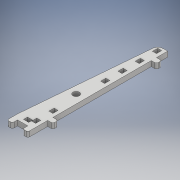
# Autodesk Inventor part: turtlebot_installation_fin_bottom
Saved by Autodesk Inventor 2018 (Build 220112000, 112)
## iProperties
Created: 2018-07-15
Part Number: turtlebot_installation_fin_bottom
Material: Generic
Document SubType Name: Modeling
Designer: Tsche
Density: 1 g/cm^3
Appearance: Default
Author: Tsche
Autodesk Inventor part; units mm, degrees
ref_plane "YZ Plane" through (0, 0, 0) normal (1, 0, 0) x (0, 1, 0)
ref_plane "XZ Plane" through (0, 0, 0) normal (0, 1, 0) x (-1, 0, 0)
ref_plane "XY Plane" through (0, 0, 0) normal (0, 0, 1) x (1, 0, 0)
sketch "Sketch1" plane through (0, 0, 0) normal (0, 0, 1) x (1, 0, 0)
  line L0 (0, 0) -> (0, 8.5)
  line L1 (0, 8.5) -> (3, 8.5)
  line L2 (3, 8.5) -> (3, 11.5)
  line L3 (3, 11.5) -> (0, 11.5)
  line L4 (0, 11.5) -> (0, 68.5)
  line L5 (0, 68.5) -> (3, 68.5)
  line L6 (3, 68.5) -> (3, 71.5)
  line L7 (3, 71.5) -> (0, 71.5)
  line L8 (0, 71.5) -> (0, 78)
  line L9 (-12, 0) -> (-12, -3)
  line L10 (-12, -3) -> (-9, -3)
  line L11 (-9, -3) -> (-9, 0)
  line L12 (-9, 0) -> (-3, 0)
  line L13 (-3, 0) -> (-3, -3)
  line L14 (-3, -3) -> (0, -3)
  line L15 (0, -3) -> (0, 0)
  line L16 (0, 78) -> (-5.5, 78)
  line L17 (-12, 0) -> (-12, 3)
  line L18 (-12, 3) -> (-5.5, 78)
  line L19 (-15, 0) -> (6, 0) construction
  line L20 (3, 10) -> (0, 10) construction
  line L21 (3, 70) -> (0, 70) construction
  line L22 (-4.3, 76.5) -> (-3, 76.5)
  line L23 (-3, 76.5) -> (-3, 73.5)
  line L24 (-3, 73.5) -> (-4.3, 73.5)
  line L25 (-4.3, 73.5) -> (-4.3, 76.5)
  line L26 (-4.3, 75) -> (-3, 75) construction
  line L27 (-7.5, 4.3) -> (-4.5, 4.3)
  line L28 (-4.5, 4.3) -> (-4.5, 3)
  line L29 (-4.5, 3) -> (-7.5, 3)
  line L30 (-7.5, 3) -> (-7.5, 4.3)
  line L31 (-6, 3) -> (-6, 0) construction
  line L32 (-4.3, 66.5) -> (-3, 66.5)
  line L33 (-3, 66.5) -> (-3, 63.5)
  line L34 (-3, 63.5) -> (-4.3, 63.5)
  line L35 (-4.3, 63.5) -> (-4.3, 66.5)
  line L36 (-4.3, 65) -> (-3, 65) construction
  line L37 (-4.3, 16.5) -> (-3, 16.5)
  line L38 (-3, 16.5) -> (-3, 13.5)
  line L39 (-3, 13.5) -> (-4.3, 13.5)
  line L40 (-4.3, 13.5) -> (-4.3, 16.5)
  line L41 (-4.3, 15) -> (-3, 15) construction
  line L42 (-3, 6.5) -> (-4.3, 6.5)
  line L43 (-4.3, 5) -> (-3, 5) construction
  line L44 (-3, 3.5) -> (-3, 6.5)
  line L45 (-4.3, 3.5) -> (-3, 3.5)
  line L46 (-4.3, 6.5) -> (-4.3, 3.5)
  line L47 (0, 50) -> (-3, 50) construction
  line L48 (-4.3, 53.5) -> (-3, 53.5)
  line L49 (-3, 53.5) -> (-3, 56.5)
  line L50 (-3, 56.5) -> (-4.3, 56.5)
  line L51 (-4.3, 56.5) -> (-4.3, 53.5)
  line L52 (-4.3, 55) -> (-3, 55) construction
  line L53 (-4.3, 46.5) -> (-3, 46.5)
  line L54 (-3, 46.5) -> (-3, 43.5)
  line L55 (-3, 43.5) -> (-4.3, 43.5)
  line L56 (-4.3, 43.5) -> (-4.3, 46.5)
  line L57 (-4.3, 45) -> (-3, 45) construction
  circle A0 centre (-5, 30) radius 1.85
  dimension "d0" = 3
  dimension "d1" = 12
  dimension "d2" = 3
  dimension "d3" = 10
  dimension "d4" = 60
  dimension "d5" = 5.5
  dimension "d6" = 3
  dimension "d7" = 1.3
  dimension "d8" = 3
  dimension "d9" = 5
  dimension "d10" = 3
  dimension "d11" = 1.3
  dimension "d12" = 3
  dimension "d13" = 3
  dimension "d14" = 3
  dimension "d15" = 1.3
  dimension "d16" = 5
  dimension "d17" = 3
  dimension "d18" = 1.3
  dimension "d19" = 5
  dimension "d29" = 5
  dimension "d30" = 50
  dimension "d31" = 3.7
  dimension "d32" = 5
  dimension "d33" = 30
  constraints: 114 end point, 16 perpendicular, 13 midpoint, 12 symmetric about line, 11 parallel, 11 point on line, 9 horizontal, 8 equal length, 4 collinear, 3 vertical, 1 centre point
  measures "d0" distance of L12.end L13.end
  measures "d1" distance between parallel lines of L15 L9
  measures "d2" distance of L9.start L17.end
  measures "d3" distance between parallel lines of L20 L19
  measures "d4" distance between parallel lines of L20 L21
  measures "d5" distance of L8.end L16.end
  measures "d6" distance of L24.end L22.start
  measures "d7" distance between parallel lines of L23 L25
  measures "d8" distance between parallel lines of L8 L23
  measures "d9" distance between parallel lines of L26 L21
  measures "d10" distance between parallel lines of L16 L26
  measures "d11" distance of L29.end L27.start
  measures "d12" distance of L28.end L29.end
  measures "d13" distance between parallel lines of L29 L12
  measures "d14" distance of L34.end L32.start
  measures "d15" distance between parallel lines of L33 L35
  measures "d16" distance between parallel lines of L36 L21
  measures "d17" distance of L39.end L37.start
  measures "d18" distance between parallel lines of L38 L40
  measures "d19" distance between parallel lines of L41 L20
  measures "d29" distance between parallel lines of L52 L47
  measures "d30" distance between parallel lines of L19 L47
  measures "d31" diameter of A0
  measures "d32" distance from line of L4 A0.centre
  measures "d33" distance from line of L19 A0.centre
extrude "Extrusion1" add sketch "Sketch1" along normal blind 3
fillet "Fillet1" radius 1 8 edges at (3, 11.5, 1.5) (3, 8.5, 1.5) (0, -3, 1.5) (-3, -3, 1.5) (-9, -3, 1.5) (-12, -3, 1.5) (3, 68.5, 1.5) (3, 71.5, 1.5)
fillet "Fillet2" radius 3 1 edges at (-5.5, 78, 1.5)
fillet "Fillet2" radius 20 1 edges at (-12, 3, 1.5)
chamfer "Chamfer1" distance 1 angle 45 14 edges at (-6, 3, 3) (-6, 3, 0) (-3, 15, 3) (-3, 15, 0) (-3, 65, 3) (-3, 65, 0) (-3, 75, 3) (-3, 75, 0) (-3, 5, 3) (-3, 5, 0) (-3, 45, 0) (-3, 45, 3) (-3, 55, 0) (-3, 55, 3)
body "Solid1"
